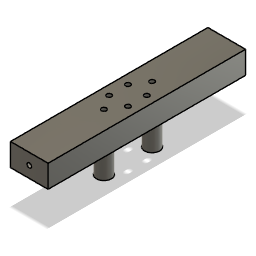
GPS+hinge stand v8 (Autodesk Fusion 360 design; units mm, degrees)
Autodesk Fusion 360 part; units mm, degrees
sketch "Sketch1" plane through (0, 0, 0) normal (0, 0, 1) x (1, 0, 0)
  line L0 (0, 0) -> (25, 0)
  line L1 (25, 0) -> (25, 15)
  line L2 (25, 15) -> (0, 15)
  line L3 (0, 15) -> (0, 0)
  dimension "d1" = 25
  dimension "d2" = 15
  constraint horizontal L0
  constraint vertical L1
  constraint horizontal L2
  constraint vertical L3
  constraint coincident L0.start L3.end
  measures "d1" distance of L0.start L0.end
  measures "d2" distance of L0.start L2.end
extrude "Extrude1" add sketch "Sketch1" along normal blind 131.11
sketch "Sketch2" plane through (0, 0, 131.11) normal (0, 0, 1) x (1, 0, 0)
  line L0 (0, 15) -> (0, 0)
  line L1 (0, 0) -> (25, 0)
  line L2 (25, 0) -> (25, 15)
  line L3 (25, 15) -> (0, 15)
  circle A0 centre (12.5, 7.5) radius 1.5
  dimension "d5" = 3
  measures "d5" diameter of A0
extrude "Extrude2" cut sketch "Sketch2" against normal blind 180 contours A0
sketch "Sketch3" plane through (0, 15, 0) normal (0, 1, 0) x (-1, 0, 0)
  line L0 (-25, 0) -> (0, 0)
  line L1 (0, 0) -> (0, 131.11)
  line L2 (0, 131.11) -> (-25, 131.11)
  line L3 (-25, 131.11) -> (-25, 0)
  circle A0 centre (-12.5, 49.555) radius 1.6
  circle A1 centre (-12.5, 81.555) radius 1.6
  dimension "d8" = 3.2
  dimension "d24" = 3.2
  measures "d8" diameter of A0
  measures "d24" diameter of A1
extrude "Extrude3" cut sketch "Sketch3" against normal blind 51 contours A0 | A1
sketch "Sketch4" plane through (0, 15, 0) normal (0, 1, 0) x (-1, 0, 0)
  circle A0 centre (-12.5, 81.555) radius 1.6
  circle A1 centre (-12.5, 49.555) radius 1.6
  line L0 (-25, 0) -> (0, 0)
  line L1 (0, 0) -> (0, 131.11)
  line L2 (0, 131.11) -> (-25, 131.11)
  line L3 (-25, 131.11) -> (-25, 0)
  line L4 (-25, 78.055) -> (0, 78.055)
  line L5 (0, 78.055) -> (0, 53.055)
  line L6 (0, 53.055) -> (-25, 53.055)
  line L7 (-25, 53.055) -> (-25, 78.055)
  line L8 (-25, 78.055) -> (0, 53.055) construction
  line L9 (0, 78.055) -> (-25, 53.055) construction
  point P0 (-12.5, 65.555)
  dimension "d12" = 25
  dimension "d13" = 25
  constraint horizontal L4
  constraint perpendicular L4 L5
  constraint parallel L4 L6
  constraint parallel L5 L7
  constraint coincident L8 P0
  constraint coincident L9 P0
  measures "d12" distance of L5.end L6.end
  measures "d13" distance of L4.end L5.end
sketch "Sketch6" plane through (0, 0, 0) normal (0, -1, 0) x (1, 0, 0)
  circle A0 centre (12.5, 81.555) radius 1.6
  circle A1 centre (12.5, 49.555) radius 1.6
  line L0 (0, 0) -> (25, 0)
  line L1 (25, 0) -> (25, 131.11)
  line L2 (25, 131.11) -> (0, 131.11)
  line L3 (0, 131.11) -> (0, 0)
  circle A2 centre (12.5, 81.555) radius 5
  circle A3 centre (12.5, 49.555) radius 5
  dimension "d20" = 10
  dimension "d21" = 10
  constraint concentric A0 A2
  constraint concentric A1 A3
  measures "d20" diameter of A2
  measures "d21" diameter of A3
extrude "Extrude6" add sketch "Sketch6" along normal blind 22.5 contours A2 | A3
sketch "Sketch7" plane through (0, 15, 0) normal (0, 1, 0) x (-1, 0, 0)
  circle A0 centre (-12.5, 81.555) radius 1.6
  circle A1 centre (-12.5, 49.555) radius 1.6
  line L0 (-25, 0) -> (0, 0)
  line L1 (0, 0) -> (0, 131.11)
  line L2 (0, 131.11) -> (-25, 131.11)
  line L3 (-25, 131.11) -> (-25, 0)
  line L4 (-25, 53.055) -> (0, 53.055)
  line L5 (0, 53.055) -> (0, 78.055)
  line L6 (0, 78.055) -> (-25, 78.055)
  line L7 (-25, 78.055) -> (-25, 53.055)
  circle A2 centre (-6.25, 59.305) radius 1.6
  circle A3 centre (-6.25, 71.805) radius 1.6
  line L8 (-12.5, 65.555) -> (-12.5, 69)
  circle A4 centre (-18.75, 59.305) radius 1.6
  circle A5 centre (-18.75, 71.805) radius 1.6
  point P0 (-12.5, 65.555)
  dimension "d25" = 25
  dimension "d26" = 25
  dimension "d27" = 3.2
  dimension "d28" = 6.25
  dimension "d29" = 6.25
  dimension "d30" = 3.2
  dimension "d31" = 12.5
  constraint horizontal L4
  constraint perpendicular L4 L5
  constraint parallel L4 L6
  constraint parallel L5 L7
  constraint coincident P0 L8.start
  constraint parallel L5 L8
  constraint symmetric A2 L8 A4
  constraint symmetric A3 L8 A5
  measures "d25" distance of L5.end L6.end
  measures "d26" distance of L4.end L5.end
  measures "d27" diameter of A2
  measures "d28" horizontal distance of P0 A2.centre
  measures "d29" distance of L4 A2.centre
  measures "d30" diameter of A3
  measures "d31" distance of A2.centre A3.centre
extrude "Extrude7" cut sketch "Sketch7" against normal blind 17 contours A2 | A3 | A4 | A5
fillet "Fillet1" radius 7.5 2 edges at (7.8384, 0, 83.3631) (7.8384, 0, 51.3631)
sketch "Sketch8" plane through (0, 0, 0) normal (0, -1, 0) x (1, 0, 0)
  arc A0 (4.6502, 59.2828) -> (0, 49.555) centre (12.5, 49.555) ccw
  arc A1 (6.9381, 60.7495) -> (4.6502, 59.2828) centre (6.25, 59.305) ccw
  arc A2 (18.0619, 60.7495) -> (6.9381, 60.7495) centre (12.5, 49.555) ccw
  arc A3 (20.3498, 59.2828) -> (18.0619, 60.7495) centre (18.75, 59.305) ccw
  arc A4 (25, 49.555) -> (20.3498, 59.2828) centre (12.5, 49.555) ccw
  line L0 (25, 49.555) -> (25, 81.555)
  arc A5 (20.3498, 71.8272) -> (25, 81.555) centre (12.5, 81.555) ccw
  arc A6 (18.0619, 70.3605) -> (20.3498, 71.8272) centre (18.75, 71.805) ccw
  arc A7 (6.9381, 70.3605) -> (18.0619, 70.3605) centre (12.5, 81.555) ccw
  arc A8 (4.6502, 71.8272) -> (6.9381, 70.3605) centre (6.25, 71.805) ccw
  arc A9 (0, 81.555) -> (4.6502, 71.8272) centre (12.5, 81.555) ccw
  line L1 (0, 81.555) -> (0, 49.555)
  circle A10 centre (6.25, 59.305) radius 3.5
  circle A11 centre (18.75, 59.305) radius 3.5
  circle A12 centre (6.25, 71.805) radius 3.5
  circle A13 centre (18.75, 71.805) radius 3.5
  dimension "d36" = 7
  dimension "d37" = 7
  dimension "d38" = 7
  dimension "d39" = 7
  constraint concentric A1 A10
  constraint concentric A3 A11
  constraint concentric A8 A12
  constraint concentric A6 A13
  measures "d36" diameter of A10
  measures "d37" diameter of A11
  measures "d38" diameter of A12
  measures "d39" diameter of A13
extrude "Extrude8" cut sketch "Sketch8" along normal blind 6 contours A0 A1 A2 A10 | A2 A3 A4 A11 | A7 A8 A9 A12 | A5 A6 A7 A13 picked at (6.5291, 58.7685) picked at (18.3538, 58.8458) picked at (6.5291, 72.3415) picked at (18.4982, 72.3568)
equation "d22 = 42.5 mm - 40 mm + 20 mm"
equation "d28 = 25 / 4 * 1 mm"
equation "d31 = 25 / 2 * 1 mm"
